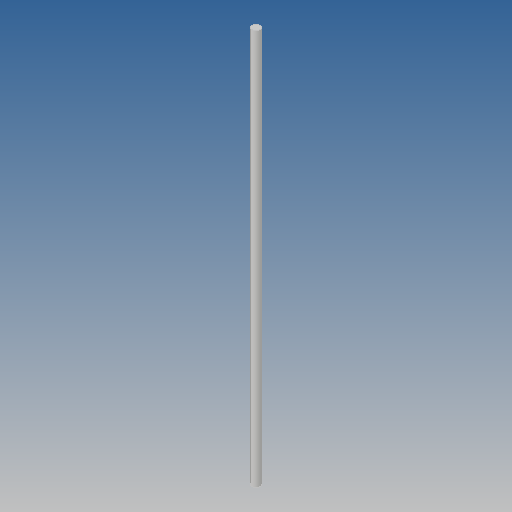
# Autodesk Inventor part: SmallRod
Saved by Autodesk Inventor 2018 (Build 220112000, 112)
## iProperties
Created: 2022-08-28
Part Number: SmallRod
Material: Generic
Document SubType Name: Modeling
Designer: Nathann
Density: 1 g/cm^3
Appearance: Default
Author: Nathann
Autodesk Inventor part; units mm, degrees
ref_plane "YZ Plane" through (0, 0, 0) normal (1, 0, 0) x (0, 1, 0)
ref_plane "XZ Plane" through (0, 0, 0) normal (0, 1, 0) x (-1, 0, 0)
ref_plane "XY Plane" through (0, 0, 0) normal (0, 0, 1) x (1, 0, 0)
sketch "Sketch1" plane through (0, 0, 0) normal (0, 1, 0) x (-1, 0, 0)
  circle A0 centre (0, 0) radius 4
  dimension "d0" = 8
  constraints: 1 centre point, 1 coincident
  measures "d0" diameter of A0
extrude "Extrusion1" add sketch "Sketch1" along normal blind 400
equation "\"d0\" = RodDiameter"
equation "\"d1\" = SmallRodLenght"
equation "\"RodDiameter\" = 8"
equation "\"SmallRodLenght\" = 400"
equation "\"VerticalBearingOD\" = 16"
equation "\"PrintingClearance\" = 0.2"
equation "\"TubeID\" = 18"
body "Solid1"
